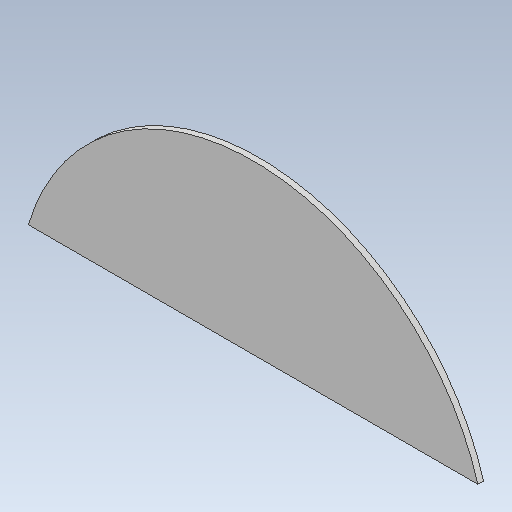
# Autodesk Inventor part: cover_side
Saved by Autodesk Inventor 2021 (Build 250183000, 183)
## iProperties
Created: 2021-05-06
Part Number: cover_side
Material: Generic
Document SubType Name: Modeling
Designer: Watchdog
Density: 1 g/cm^3
Appearance: Default
Author: Watchdog
Autodesk Inventor part; units mm, degrees
ref_plane "YZ Plane" through (0, 0, 0) normal (1, 0, 0) x (0, 1, 0)
ref_plane "XZ Plane" through (0, 0, 0) normal (0, 1, 0) x (-1, 0, 0)
ref_plane "XY Plane" through (0, 0, 0) normal (0, 0, 1) x (1, 0, 0)
sketch "Sketch2" plane through (0, 0, 0) normal (0, 0, 1) x (1, 0, 0)
  arc A0 (790, 0) -> (-790, 0) centre (0, -233.8983) ccw
  line L0 (-790, 0) -> (790, 0)
  point P0 (0, 0)
  point P1 (0, 590)
  dimension "d17" = 0
  dimension "d21" = 0
  dimension "d24" = 590
  dimension "d25" = 1580
  dimension "d26" = 790
  constraints: 3 point on circle, 2 end point, 1 centre point, 1 horizontal
  measures "d17" horizontal distance of point (0, 0) point (0, 590)
  measures "d21" vertical distance of point (0, 0) L0.start
  measures "d24" distance of point (0, 0) point (0, 590)
  measures "d25" distance of L0.end L0.start
  measures "d26" distance of point (0, 0) L0.start
extrude "side" add sketch "Sketch2" along normal blind 20
equation "\"d24\" = cover_height_main - cover_shell_thickness"
equation "\"d25\" = cover_length_main - 2 * cover_shell_thickness"
equation "\"d26\" = 0.5 * d25"
equation "\"d14\" = cover_side_thickness"
equation "\"cover_height_main\" = 600"
equation "\"cover_shell_thickness\" = 10"
equation "\"rack_tooth_thickness\" = 5"
equation "\"rack_tooth_addendum\" = 5"
equation "\"rack_tooth_dedendum\" = 5"
equation "\"cover_side_thickness\" = 20"
equation "\"cover_length_main\" = 1600"
body "Solid2"
